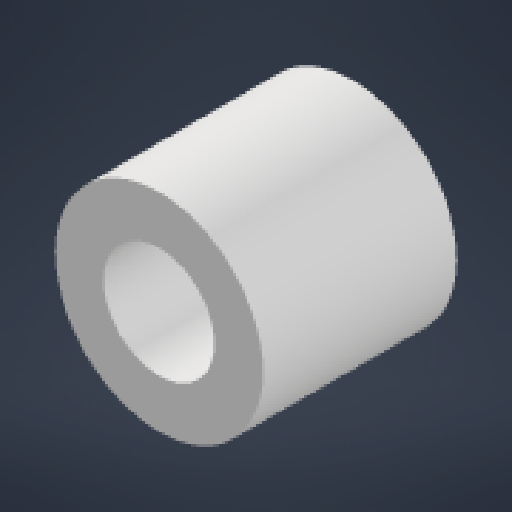
# Autodesk Inventor part: claw_spacer
Saved by Autodesk Inventor 2026 (Build 300175000, 175)
## iProperties
Created: 2025-03-27
Part Number: claw_spacer
Material: Generic
Document SubType Name: Modeling
Designer: paris
Density: 1 g/cm^3
Appearance: Default
Author: paris
Autodesk Inventor part; units mm, degrees
ref_plane "YZ Plane" through (0, 0, 0) normal (1, 0, 0) x (0, 1, 0)
ref_plane "XZ Plane" through (0, 0, 0) normal (0, 1, 0) x (-1, 0, 0)
ref_plane "XY Plane" through (0, 0, 0) normal (0, 0, 1) x (1, 0, 0)
sketch "Sketch1" plane through (0, 0, 0) normal (0, 0, 1) x (1, 0, 0)
  line L0 (-19.6493, 54.0192) -> (-19.6493, 51.5192) projected
  line L1 (-19.6493, 51.5192) -> (-17.1493, 50.3535) projected
  line L2 (-17.1493, 50.3535) -> (-17.1493, 47.8535) projected
  line L3 (-17.1493, 47.8535) -> (-19.6493, 46.6877) projected
  line L4 (-19.6493, 46.6877) -> (-19.6493, 44.1877) projected
  line L5 (-19.6493, 44.1877) -> (-17.1493, 43.0219) projected
  line L6 (-17.1493, 43.0219) -> (-17.1493, 40.5219) projected
  line L7 (-17.1493, 40.5219) -> (-19.6493, 39.3562) projected
  line L8 (-19.6493, 39.3562) -> (-19.6493, 36.8562) projected
  line L9 (-19.6493, 36.8562) -> (-17.1493, 35.6904) projected
  line L10 (-17.1493, 35.6904) -> (-17.1493, 33.1904) projected
  line L11 (-17.1493, 33.1904) -> (-19.6493, 32.0246) projected
  line L12 (-19.6493, 32.0246) -> (-19.6493, 29.5246) projected
  line L13 (-19.6493, 29.5246) -> (-17.1493, 28.3588) projected
  line L14 (-17.1493, 28.3588) -> (-17.1493, 27.685) projected
  arc A0 (-17.1493, 27.685) -> (-16.1428, 26.9802) centre (-16.3993, 27.685) ccw projected
  line L15 (-16.1428, 26.9802) -> (-10.6172, 28.9914) projected
  line L16 (-10.6172, 28.9914) -> (10.596, 7.7782) projected
  line L17 (10.596, 7.7782) -> (10.596, -7.2218) projected
  line L18 (10.596, -7.2218) -> (-10.6172, -28.435) projected
  line L19 (-10.6172, -28.435) -> (-10.6172, -58.435) projected
  line L20 (-10.6172, -58.435) -> (-0.6172, -58.435) projected
  line L21 (-0.6172, -58.435) -> (-0.6172, -33.435) projected
  line L22 (-0.6172, -33.435) -> (18.096, -14.7218) projected
  arc A1 (18.096, -14.7218) -> (19.6493, -10.9718) centre (14.346, -10.9718) ccw projected
  line L23 (19.6493, -10.9718) -> (19.6493, 11.5282) projected
  arc A2 (19.6493, 11.5282) -> (18.096, 15.2782) centre (14.346, 11.5282) ccw projected
  line L24 (18.096, 15.2782) -> (-10.6172, 43.9914) projected
  line L25 (-10.6172, 43.9914) -> (-15.6946, 57.9415) projected
  arc A3 (-15.6946, 57.9415) -> (-17.1493, 57.685) centre (-16.3993, 57.685) ccw projected
  line L26 (-17.1493, 57.685) -> (-17.1493, 55.185) projected
  line L27 (-17.1493, 55.185) -> (-19.6493, 54.0192) projected
  circle A4 centre (-5.6172, -50.935) radius 2 projected
  circle A5 centre (-5.6172, -35.935) radius 2 projected
  circle A6 centre (14.346, 11.5282) radius 2 projected
  circle A7 centre (14.346, -10.9718) radius 2 projected
  circle A8 centre (-10.6172, 36.4914) radius 2 projected
  circle A9 centre (-10.6172, 36.4914) radius 3.75
  point P0 (0, 0)
  dimension "d0" = 7.5
  constraints: 1 centre point, 1 coincident
  measures "d0" diameter of A9
extrude "Extrusion1" add sketch "Sketch1" along normal blind 7 contours A9
body "Solid1"
